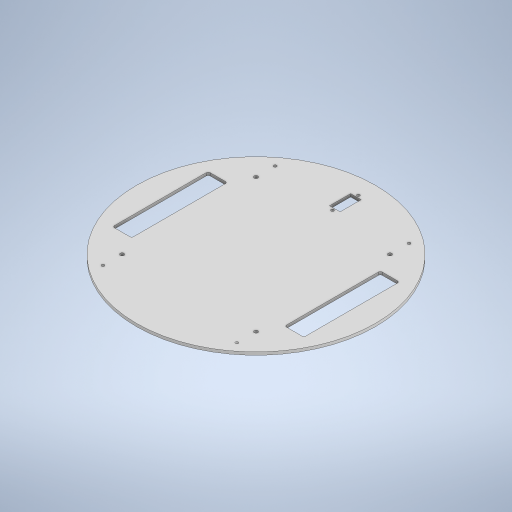
# Autodesk Inventor part: Part2
Saved by Autodesk Inventor 2023.3 (Build 273359000, 359)
## iProperties
Created: 2023-08-25
Part Number: Part2
Material: Generic
Document SubType Name: Modeling
Designer: husse
Density: 1 g/cm^3
Appearance: Default
Author: husse
Autodesk Inventor part; units mm, degrees
ref_plane "YZ Plane" through (0, 0, 0) normal (1, 0, 0) x (0, 1, 0)
ref_plane "XZ Plane" through (0, 0, 0) normal (0, 1, 0) x (-1, 0, 0)
ref_plane "XY Plane" through (0, 0, 0) normal (0, 0, 1) x (1, 0, 0)
sketch "Sketch1" plane through (0, 0, 0) normal (0, 1, 0) x (-1, 0, 0)
  circle A0 centre (0, 0) radius 125
  circle A1 centre (70, -90) radius 1.5
  circle A2 centre (-70, -90) radius 1.5
  circle A3 centre (-70, 90) radius 1.5
  circle A4 centre (70, 90) radius 1.5
  circle A5 centre (70, -70) radius 2
  circle A6 centre (-70, -70) radius 2
  circle A7 centre (-70, 70) radius 2
  circle A8 centre (70, 70) radius 2
  line L0 (5, -104.4418) -> (-5.5, -104.4418)
  line L1 (-5.5, -82.9418) -> (-5.5, -104.4418)
  line L2 (-5, -82.4418) -> (5.5, -82.4418)
  line L3 (5.5, -103.9418) -> (5.5, -82.4418)
  line L4 (-5, -82.4418) -> (-5.5, -82.4418)
  line L5 (-5.5, -82.4418) -> (-5.5, -82.9418)
  line L6 (5.5, -103.9418) -> (5.5, -104.4418)
  line L7 (5.5, -104.4418) -> (5, -104.4418)
  arc A9 (0.75, -108.2408) -> (-0.75, -108.2408) centre (0, -106.9418) ccw
  arc A10 (-0.75, -78.6427) -> (0.75, -78.6427) centre (0, -79.9418) ccw
  circle A11 centre (0, -106.9418) radius 1.5
  circle A12 centre (0, -79.9418) radius 1.5
  line L8 (98, 50) -> (82, 50)
  line L9 (80, 48) -> (80, -48)
  line L10 (82, -50) -> (98, -50)
  line L11 (100, -48) -> (100, 48)
  line L12 (-98, 50) -> (-82, 50)
  line L13 (-80, 48) -> (-80, -48)
  line L14 (-82, -50) -> (-98, -50)
  line L15 (-100, -48) -> (-100, 48)
  arc A13 (98, -50) -> (100, -48) centre (98, -48) ccw
  arc A14 (100, 48) -> (98, 50) centre (98, 48) ccw
  arc A15 (82, 50) -> (80, 48) centre (82, 48) ccw
  arc A16 (80, -48) -> (82, -50) centre (82, -48) ccw
  arc A17 (-82, -50) -> (-80, -48) centre (-82, -48) ccw
  arc A18 (-80, 48) -> (-82, 50) centre (-82, 48) ccw
  arc A19 (-98, 50) -> (-100, 48) centre (-98, 48) ccw
  arc A20 (-100, -48) -> (-98, -50) centre (-98, -48) ccw
  point P0 (0.75, -108.2408)
  point P1 (-0.75, -78.6427)
  point P2 (0.75, -78.6427)
  point P3 (-90, 0)
  constraints: 32 end point, 20 centre point, 20 point on circle, 16 tangent, 12 horizontal, 10 vertical, 7 equal radius, 3 coincident, 2 collinear, 2 parallel, 1 perpendicular, 70 other
extrude "Extrusion6" add sketch "Sketch1" along normal blind 3
body "Solid6"
